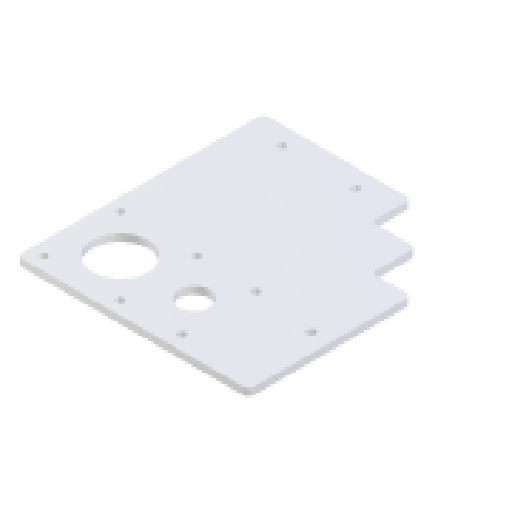
# Autodesk Inventor part: Z Axis Motor Mount
Saved by Autodesk Inventor 2023.2 (Build 272271000, 271)
## iProperties
Created: 2023-02-02
Part Number: Z Axis Motor Mount
Material: Aluminum 6061
Document SubType Name: Modeling
Designer: remop
Density: 2.7 g/cm^3
Appearance: Aluminum - Flat
Author: remop
Autodesk Inventor part; units mm, degrees
ref_plane "YZ Plane" through (0, 0, 0) normal (1, 0, 0) x (0, 1, 0)
ref_plane "XZ Plane" through (0, 0, 0) normal (0, 1, 0) x (-1, 0, 0)
ref_plane "XY Plane" through (0, 0, 0) normal (0, 0, 1) x (1, 0, 0)
sketch "Sketch1" plane through (0, 0, 0) normal (0, 1, 0) x (-1, 0, 0)
  line L0 (0, 34) -> (0, 100)
  line L1 (0, 100) -> (94, 100)
  line L2 (94, 100) -> (94, 0)
  line L3 (94, 0) -> (34, 0)
  circle A0 centre (57.5, 94.5) radius 1.6
  circle A1 centre (88.5, 94.5) radius 1.6
  circle A2 centre (88.5, 63.5) radius 1.6
  circle A3 centre (57.5, 63.5) radius 1.6
  circle A4 centre (73, 79) radius 11.25
  circle A5 centre (43, 79) radius 6.25
  line L4 (34, 16) -> (16, 16)
  line L5 (16, 16) -> (16, 34)
  line L6 (34, 0) -> (34, 16)
  line L7 (16, 34) -> (0, 34)
  circle A6 centre (33, 64) radius 1.6
  circle A7 centre (33, 94) radius 1.6
  point P0 (0, 0)
  dimension "d3" = 100
  dimension "d4" = 60
  dimension "d5" = 31
  dimension "d6" = 31
  dimension "d7" = 15.5
  dimension "d8" = 15.5
  dimension "d9" = 22.5
  dimension "d10" = 21
  dimension "d11" = 12.5
  dimension "d12" = 21
  dimension "d13" = 3.2
  dimension "d14" = 30
  dimension "d15" = 16
  dimension "d16" = 34
  dimension "d17" = 34
  dimension "d18" = 15
  dimension "d19" = 15
  dimension "d20" = 10
  constraints: 16 end point, 8 centre point, 5 equal radius, 5 perpendicular, 4 horizontal alignment, 4 vertical alignment, 2 horizontal, 2 vertical
  measures "d3" distance between parallel lines of L1 L3
  measures "d4" distance of L2.end L3.end
  measures "d5" distance of A1.centre A0.centre
  measures "d6" distance of A3.centre A0.centre
  measures "d7" horizontal distance of A4.centre A0.centre
  measures "d8" horizontal distance of A1.centre A4.centre
  measures "d9" diameter of A4
  measures "d10" distance from line of L1 A4.centre
  measures "d11" diameter of A5
  measures "d12" distance from line of L2 A4.centre
  measures "d13" diameter of A0
  measures "d14" distance of A4.centre A5.centre
  measures "d15" distance between parallel lines of L3 L4
  measures "d16" distance between parallel lines of L7 L3
  measures "d17" distance between parallel lines of L0 L6
  measures "d18" vertical distance of A6.centre A5.centre
  measures "d19" vertical distance of A7.centre A5.centre
  measures "d20" horizontal distance of A5.centre A7.centre
extrude "Extrusion1" add sketch "Sketch1" along normal blind 3
fillet "Fillet1" radius 2 8 edges at (-16, 1.5, 34) (-34, 1.5, 16) (-16, 1.5, 16) (0, 1.5, 34) (-34, 1.5, 0) (0, 1.5, 100) (-94, 1.5, 100) (-94, 1.5, 0)
sketch "Sketch2" plane through (0, 0, 0) normal (0, -1, 0) x (1, 0, 0)
  arc A0 (-94, 2) -> (-92, 0) centre (-92, 2) ccw projected
  line L0 (-36, 0) -> (-92, 0) projected
  arc A1 (-36, 0) -> (-34, 2) centre (-36, 2) ccw projected
  line L1 (-34, 14) -> (-34, 2) projected
  arc A2 (-32, 16) -> (-34, 14) centre (-32, 14) ccw projected
  line L2 (-18, 16) -> (-32, 16) projected
  arc A3 (-18, 16) -> (-16, 18) centre (-18, 18) ccw projected
  line L3 (-16, 32) -> (-16, 18) projected
  arc A4 (-14, 34) -> (-16, 32) centre (-14, 32) ccw projected
  line L4 (-2, 34) -> (-14, 34) projected
  arc A5 (-2, 34) -> (0, 36) centre (-2, 36) ccw projected
  line L5 (0, 98) -> (0, 36) projected
  arc A6 (0, 98) -> (-2, 100) centre (-2, 98) ccw projected
  line L6 (-92, 100) -> (-2, 100) projected
  arc A7 (-92, 100) -> (-94, 98) centre (-92, 98) ccw projected
  line L7 (-94, 2) -> (-94, 98) projected
  circle A8 centre (-33, 94) radius 1.6 projected
  circle A9 centre (-33, 64) radius 1.6 projected
  circle A10 centre (-43, 79) radius 6.25 projected
  circle A11 centre (-73, 79) radius 11.25 projected
  circle A12 centre (-57.5, 63.5) radius 1.6 projected
  circle A13 centre (-88.5, 63.5) radius 1.6 projected
  circle A14 centre (-88.5, 94.5) radius 1.6 projected
  circle A15 centre (-57.5, 94.5) radius 1.6 projected
  point P0 (0, 0)
  point P1 (-7.5, 67)
  point P2 (-49, 7.5)
  point P3 (-79, 7.5)
  point P4 (0, 67)
  dimension "d22" = 7.5
  dimension "d23" = 7.5
  dimension "d24" = 15
  dimension "d25" = 15
  constraints: 2 horizontal alignment, 1 midpoint
  measures "d22" distance from line of L5 point (-7.5, 67)
  measures "d23" distance from line of L0 point (-49, 7.5)
  measures "d24" distance from line of L1 point (-49, 7.5)
  measures "d25" distance from line of L7 point (-79, 7.5)
hole "Hole1" at (-7.5, 0, 67) at (-49, 0, 7.5) at (-79, 0, 7.5) direction (0, 1, 0) diameter 3.4 end through all clearance for "Countersunk Flat Head Screw ISO 2009/7046" size "M3" standard "ISO"
equation "\"d6\" = d5"
equation "\"d7\" = 0.5 * d6"
equation "\"d8\" = 0.5 * d5"
equation "\"d19\" = d18"
equation "\"d23\" = d22"
equation "\"d25\" = d24"
body "Solid1"
